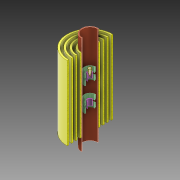
# Autodesk Inventor part: DemoCrossSect
Saved by Autodesk Inventor 2021 (Build 250183000, 183)
## iProperties
Created: 2023-01-16
Part Number: DemoCrossSect
Material: Copper
Document SubType Name: Modeling
Designer: Eli
Density: 8.94 g/cm^3
Appearance: Copper - Satin
Author: Eli
Autodesk Inventor part; units mm, degrees
ref_plane "YZ Plane" through (0, 0, 0) normal (1, 0, 0) x (0, 1, 0)
ref_plane "XZ Plane" through (0, 0, 0) normal (0, 1, 0) x (-1, 0, 0)
ref_plane "XY Plane" through (0, 0, 0) normal (0, 0, 1) x (1, 0, 0)
sketch "Sketch1" plane through (0, 0, 0) normal (0, 0, 1) x (1, 0, 0)
  line L0 (18.1725, 115.942) -> (19.9396, 115.942)
  line L1 (19.9396, 115.942) -> (19.9396, 77.2947)
  line L2 (19.9396, -115.942) -> (18.1725, -115.942)
  line L3 (18.1725, -115.942) -> (18.1725, 115.942)
  line L4 (19.9396, 77.2947) -> (19.9396, -77.2947)
  line L5 (19.9396, -77.2947) -> (19.9396, -115.942)
  line L6 (27.9401, -86.9565) -> (30.8386, -86.9565)
  line L7 (0, 289.8551) -> (0, -289.8551)
  line L8 (0, 57.971) -> (0, -57.971)
  line L9 (5.314, 35.2657) -> (6.2802, 35.2657)
  line L10 (5.314, 20.7729) -> (6.2802, 20.7729)
  line L11 (5.314, 35.2657) -> (5.314, 20.7729)
  line L12 (6.2802, 20.7729) -> (6.2802, 35.2657)
  arc A0 (0, -289.8551) -> (0, 289.8551) centre (0, 0) ccw
  arc A1 (9.6618, 30.9179) -> (11.6908, 30.9179) centre (10.6763, 30.9179) ccw
  arc A2 (11.6908, 30.9179) -> (9.6618, 30.9179) centre (10.6763, 30.9179) ccw
  arc A3 (9.6618, 32.9952) -> (11.6908, 32.9952) centre (10.6763, 32.9952) ccw
  arc A4 (11.6908, 32.9952) -> (9.6618, 32.9952) centre (10.6763, 32.9952) ccw
  arc A5 (9.6618, 35.0725) -> (11.6908, 35.0725) centre (10.6763, 35.0725) ccw
  arc A6 (11.6908, 35.0725) -> (9.6618, 35.0725) centre (10.6763, 35.0725) ccw
  arc A7 (9.6618, 37.1498) -> (11.6908, 37.1498) centre (10.6763, 37.1498) ccw
  arc A8 (11.6908, 37.1498) -> (9.6618, 37.1498) centre (10.6763, 37.1498) ccw
  arc A9 (9.6618, 39.2271) -> (11.6908, 39.2271) centre (10.6763, 39.2271) ccw
  arc A10 (11.6908, 39.2271) -> (9.6618, 39.2271) centre (10.6763, 39.2271) ccw
  arc A11 (9.6618, 41.3043) -> (11.6908, 41.3043) centre (10.6763, 41.3043) ccw
  arc A12 (11.6908, 41.3043) -> (9.6618, 41.3043) centre (10.6763, 41.3043) ccw
  arc A13 (11.4976, 31.9614) -> (13.5266, 31.9614) centre (12.5121, 31.9614) ccw
  arc A14 (13.5266, 31.9614) -> (11.4976, 31.9614) centre (12.5121, 31.9614) ccw
  arc A15 (11.4976, 34.0386) -> (13.5266, 34.0386) centre (12.5121, 34.0386) ccw
  arc A16 (13.5266, 34.0386) -> (11.4976, 34.0386) centre (12.5121, 34.0386) ccw
  arc A17 (11.4976, 36.1159) -> (13.5266, 36.1159) centre (12.5121, 36.1159) ccw
  arc A18 (13.5266, 36.1159) -> (11.4976, 36.1159) centre (12.5121, 36.1159) ccw
  arc A19 (11.4976, 38.1932) -> (13.5266, 38.1932) centre (12.5121, 38.1932) ccw
  arc A20 (13.5266, 38.1932) -> (11.4976, 38.1932) centre (12.5121, 38.1932) ccw
  arc A21 (11.4976, 40.2705) -> (13.5266, 40.2705) centre (12.5121, 40.2705) ccw
  arc A22 (13.5266, 40.2705) -> (11.4976, 40.2705) centre (12.5121, 40.2705) ccw
  arc A23 (11.6908, 25.1208) -> (9.6618, 25.1208) centre (10.6763, 25.1208) ccw
  arc A24 (9.6618, 25.1208) -> (11.6908, 25.1208) centre (10.6763, 25.1208) ccw
  arc A25 (11.6908, 23.0435) -> (9.6618, 23.0435) centre (10.6763, 23.0435) ccw
  arc A26 (9.6618, 23.0435) -> (11.6908, 23.0435) centre (10.6763, 23.0435) ccw
  arc A27 (11.6908, 20.9662) -> (9.6618, 20.9662) centre (10.6763, 20.9662) ccw
  arc A28 (9.6618, 20.9662) -> (11.6908, 20.9662) centre (10.6763, 20.9662) ccw
  arc A29 (11.6908, 18.8889) -> (9.6618, 18.8889) centre (10.6763, 18.8889) ccw
  arc A30 (9.6618, 18.8889) -> (11.6908, 18.8889) centre (10.6763, 18.8889) ccw
  arc A31 (11.6908, 16.8116) -> (9.6618, 16.8116) centre (10.6763, 16.8116) ccw
  arc A32 (9.6618, 16.8116) -> (11.6908, 16.8116) centre (10.6763, 16.8116) ccw
  arc A33 (11.6908, 14.7343) -> (9.6618, 14.7343) centre (10.6763, 14.7343) ccw
  arc A34 (9.6618, 14.7343) -> (11.6908, 14.7343) centre (10.6763, 14.7343) ccw
  arc A35 (13.5266, 24.0773) -> (11.4976, 24.0773) centre (12.5121, 24.0773) ccw
  arc A36 (11.4976, 24.0773) -> (13.5266, 24.0773) centre (12.5121, 24.0773) ccw
  arc A37 (13.5266, 22) -> (11.4976, 22) centre (12.5121, 22) ccw
  arc A38 (11.4976, 22) -> (13.5266, 22) centre (12.5121, 22) ccw
  arc A39 (13.5266, 19.9227) -> (11.4976, 19.9227) centre (12.5121, 19.9227) ccw
  arc A40 (11.4976, 19.9227) -> (13.5266, 19.9227) centre (12.5121, 19.9227) ccw
  arc A41 (13.5266, 17.8454) -> (11.4976, 17.8454) centre (12.5121, 17.8454) ccw
  arc A42 (11.4976, 17.8454) -> (13.5266, 17.8454) centre (12.5121, 17.8454) ccw
  arc A43 (13.5266, 15.7681) -> (11.4976, 15.7681) centre (12.5121, 15.7681) ccw
  arc A44 (11.4976, 15.7681) -> (13.5266, 15.7681) centre (12.5121, 15.7681) ccw
  arc A45 (11.6908, -30.9179) -> (9.6618, -30.9179) centre (10.6763, -30.9179) ccw
  arc A46 (9.6618, -30.9179) -> (11.6908, -30.9179) centre (10.6763, -30.9179) ccw
  arc A47 (11.6908, -32.9952) -> (9.6618, -32.9952) centre (10.6763, -32.9952) ccw
  arc A48 (9.6618, -32.9952) -> (11.6908, -32.9952) centre (10.6763, -32.9952) ccw
  arc A49 (11.6908, -35.0725) -> (9.6618, -35.0725) centre (10.6763, -35.0725) ccw
  arc A50 (9.6618, -35.0725) -> (11.6908, -35.0725) centre (10.6763, -35.0725) ccw
  arc A51 (11.6908, -37.1498) -> (9.6618, -37.1498) centre (10.6763, -37.1498) ccw
  arc A52 (9.6618, -37.1498) -> (11.6908, -37.1498) centre (10.6763, -37.1498) ccw
  arc A53 (11.6908, -39.2271) -> (9.6618, -39.2271) centre (10.6763, -39.2271) ccw
  arc A54 (9.6618, -39.2271) -> (11.6908, -39.2271) centre (10.6763, -39.2271) ccw
  arc A55 (11.6908, -41.3043) -> (9.6618, -41.3043) centre (10.6763, -41.3043) ccw
  arc A56 (9.6618, -41.3043) -> (11.6908, -41.3043) centre (10.6763, -41.3043) ccw
  arc A57 (13.5266, -31.9614) -> (11.4976, -31.9614) centre (12.5121, -31.9614) ccw
  arc A58 (11.4976, -31.9614) -> (13.5266, -31.9614) centre (12.5121, -31.9614) ccw
  arc A59 (13.5266, -34.0386) -> (11.4976, -34.0386) centre (12.5121, -34.0386) ccw
  arc A60 (11.4976, -34.0386) -> (13.5266, -34.0386) centre (12.5121, -34.0386) ccw
  arc A61 (13.5266, -36.1159) -> (11.4976, -36.1159) centre (12.5121, -36.1159) ccw
  arc A62 (11.4976, -36.1159) -> (13.5266, -36.1159) centre (12.5121, -36.1159) ccw
  arc A63 (13.5266, -38.1932) -> (11.4976, -38.1932) centre (12.5121, -38.1932) ccw
  arc A64 (11.4976, -38.1932) -> (13.5266, -38.1932) centre (12.5121, -38.1932) ccw
  arc A65 (13.5266, -40.2705) -> (11.4976, -40.2705) centre (12.5121, -40.2705) ccw
  arc A66 (11.4976, -40.2705) -> (13.5266, -40.2705) centre (12.5121, -40.2705) ccw
  arc A67 (9.6618, -25.1208) -> (11.6908, -25.1208) centre (10.6763, -25.1208) ccw
  arc A68 (11.6908, -25.1208) -> (9.6618, -25.1208) centre (10.6763, -25.1208) ccw
  arc A69 (9.6618, -23.0435) -> (11.6908, -23.0435) centre (10.6763, -23.0435) ccw
  arc A70 (11.6908, -23.0435) -> (9.6618, -23.0435) centre (10.6763, -23.0435) ccw
  arc A71 (9.6618, -20.9662) -> (11.6908, -20.9662) centre (10.6763, -20.9662) ccw
  arc A72 (11.6908, -20.9662) -> (9.6618, -20.9662) centre (10.6763, -20.9662) ccw
  arc A73 (9.6618, -18.8889) -> (11.6908, -18.8889) centre (10.6763, -18.8889) ccw
  arc A74 (11.6908, -18.8889) -> (9.6618, -18.8889) centre (10.6763, -18.8889) ccw
  arc A75 (9.6618, -16.8116) -> (11.6908, -16.8116) centre (10.6763, -16.8116) ccw
  arc A76 (11.6908, -16.8116) -> (9.6618, -16.8116) centre (10.6763, -16.8116) ccw
  arc A77 (9.6618, -14.7343) -> (11.6908, -14.7343) centre (10.6763, -14.7343) ccw
  arc A78 (11.6908, -14.7343) -> (9.6618, -14.7343) centre (10.6763, -14.7343) ccw
  arc A79 (11.4976, -24.0773) -> (13.5266, -24.0773) centre (12.5121, -24.0773) ccw
  arc A80 (13.5266, -24.0773) -> (11.4976, -24.0773) centre (12.5121, -24.0773) ccw
  arc A81 (11.4976, -22) -> (13.5266, -22) centre (12.5121, -22) ccw
  arc A82 (13.5266, -22) -> (11.4976, -22) centre (12.5121, -22) ccw
  arc A83 (11.4976, -19.9227) -> (13.5266, -19.9227) centre (12.5121, -19.9227) ccw
  arc A84 (13.5266, -19.9227) -> (11.4976, -19.9227) centre (12.5121, -19.9227) ccw
  arc A85 (11.4976, -17.8454) -> (13.5266, -17.8454) centre (12.5121, -17.8454) ccw
  arc A86 (13.5266, -17.8454) -> (11.4976, -17.8454) centre (12.5121, -17.8454) ccw
  arc A87 (11.4976, -15.7681) -> (13.5266, -15.7681) centre (12.5121, -15.7681) ccw
  arc A88 (13.5266, -15.7681) -> (11.4976, -15.7681) centre (12.5121, -15.7681) ccw
  line L13 (19.9396, 86.9565) -> (23.9396, 86.9565)
  line L14 (23.9396, 86.9565) -> (23.9396, -86.9565)
  line L15 (23.9396, -86.9565) -> (19.9396, -86.9565)
  line L16 (19.9396, -86.9565) -> (19.9396, 86.9565)
  line L17 (29.9396, 86.9565) -> (33.9396, 86.9565)
  line L18 (29.9396, -86.9565) -> (29.9396, 86.9565)
  line L19 (33.9396, 86.9565) -> (33.9396, -86.9565)
  line L20 (33.9396, -86.9565) -> (29.9396, -86.9565)
  line L21 (39.9396, 86.9565) -> (43.9396, 86.9565)
  line L22 (39.9396, -86.9565) -> (39.9396, 86.9565)
  line L23 (43.9396, 86.9565) -> (43.9396, -86.9565)
  line L24 (43.9396, -86.9565) -> (39.9396, -86.9565)
  line L25 (49.9396, 86.9565) -> (53.9396, 86.9565)
  line L26 (49.9396, -86.9565) -> (49.9396, 86.9565)
  line L27 (53.9396, 86.9565) -> (53.9396, -86.9565)
  line L28 (53.9396, -86.9565) -> (49.9396, -86.9565)
  line L29 (0, 23.6243) -> (4, 38.6243)
  line L30 (4, 38.6243) -> (4, 44.6243)
  line L31 (4, 44.6243) -> (0, 44.6243)
  line L32 (0, 23.6243) -> (0, 44.6243)
  line L33 (0, -405.7971) -> (0, 405.7971) projected
  line L34 (1.1854, 28.0696) -> (0, 28.0696) construction
  arc A89 (0, 28.0696) -> (1.4909, 29.215) centre (0, 29.6126) ccw
  point P0 (9.6618, 41.3043)
  point P1 (11.6908, 41.3043)
  point P2 (11.4976, 40.2705)
  point P3 (13.5266, 40.2705)
  point P4 (9.6618, 39.2271)
  point P5 (11.6908, 39.2271)
  point P6 (11.4976, 38.1932)
  point P7 (13.5266, 38.1932)
  point P8 (9.6618, 37.1498)
  point P9 (11.6908, 37.1498)
  point P10 (9.6618, 35.0725)
  point P11 (11.6908, 35.0725)
  point P12 (11.4976, 36.1159)
  point P13 (13.5266, 36.1159)
  point P14 (11.4976, 34.0386)
  point P15 (13.5266, 34.0386)
  point P16 (9.6618, 32.9952)
  point P17 (11.6908, 32.9952)
  point P18 (11.4976, 31.9614)
  point P19 (13.5266, 31.9614)
  point P20 (9.6618, 30.9179)
  point P21 (11.6908, 30.9179)
  point P22 (11.6908, 25.1208)
  point P23 (9.6618, 25.1208)
  point P24 (13.5266, 24.0773)
  point P25 (11.4976, 24.0773)
  point P26 (11.6908, 23.0435)
  point P27 (9.6618, 23.0435)
  point P28 (13.5266, 22)
  point P29 (11.4976, 22)
  point P30 (11.6908, 20.9662)
  point P31 (9.6618, 20.9662)
  point P32 (13.5266, 19.9227)
  point P33 (11.4976, 19.9227)
  point P34 (11.6908, 18.8889)
  point P35 (9.6618, 18.8889)
  point P36 (13.5266, 17.8454)
  point P37 (11.4976, 17.8454)
  point P38 (11.6908, 16.8116)
  point P39 (9.6618, 16.8116)
  point P40 (13.5266, 15.7681)
  point P41 (11.4976, 15.7681)
  point P42 (11.6908, 14.7343)
  point P43 (9.6618, 14.7343)
  point P44 (0, 44.6243)
  point P45 (0, 23.6243)
  point P46 (0, 28.0696)
  dimension "d3" = 4
  dimension "d6" = 10
  dimension "d12" = 4
  dimension "d13" = 15
  dimension "d14" = 6
  constraints: 180 point on circle, 90 centre point, 68 end point, 6 point on line, 3 collinear, 3 perpendicular, 2 horizontal, 2 parallel, 2 tangent, 1 vertical, 23 other
  measures "d3" distance of L14.end L15.end
  measures "d6" distance of L13.start L17.start
  measures "d12" distance between parallel lines of L8 L30
  measures "d13" vertical distance of L29.start L29.end
  measures "d14" distance of L29.end L30.end
revolve "Revolution1" add sketch "Sketch1" angle 360 about axis through (0, 289.8551, 0) along (0, -1, 0) contours A2 A1 | A4 A3 | A6 A5 | A8 A7 | A10 A9 | A12 A11 | A14 A13 | A16 A15 | A18 A17 | A20 A19 | A22 A21 | A24 A23 | A26 A25 | A28 A27 | A30 A29 | A32 A31 | A34 A33 | A36 A35 | A38 A37 | A40 A39 | A42 A41 | A44 A43
revolve "Revolution2" add sketch "Sketch1" angle 360 about axis through (0, 57.971, 0) along (0, -1, 0) separate body contours L9 L12 L10 L11
revolve "Revolution3" add sketch "Sketch1" angle 360 about axis through (0, 57.971, 0) along (0, -1, 0) separate body contours L0 L1 L4 L5 L2 L3
revolve "Revolution4" add sketch "Sketch1" angle 360 about axis through (0, 289.8551, 0) along (0, -1, 0) separate body contours L13 L14 L15 L5 L4 L1 | L18 L17 L19 L20 L6 | L21 L23 L24 L22 | L25 L27 L28 L26
mirror "Mirror1" about plane through (0, 0, 0) normal (0, 1, 0) bodies 2 1
revolve "Revolution5" add sketch "Sketch1" angle 360 about axis through (0, -10, 0) along (0, 1, 0) separate body contours L31 L30 L29 A89 L7
shell "Shell1" thickness 0.25 removed faces 1 at (0.998, 44.6243, -0.8842) bodies 5
sketch "Sketch2" plane through (0, 0, 0) normal (0, 0, 1) x (1, 0, 0)
  line L0 (-4, 44.6243) -> (-4, 38.6243) projected
  line L1 (-4, 38.6243) -> (-1.4909, 29.215) projected
  arc A0 (-1.2493, 29.2794) -> (1.2493, 29.2794) centre (0, 29.6126) ccw projected
  line L2 (-3.75, 38.657) -> (-1.2493, 29.2794) projected
  line L3 (3.75, 38.657) -> (1.2493, 29.2794) projected
  line L4 (0, 28.3196) -> (0, 30.173)
  line L5 (0, 30.173) -> (1.4876, 30.173)
  point P0 (0, 0)
  constraints: 4 end point, 1 perpendicular, 1 point on circle, 1 point on line, 1 vertical
revolve "Revolution6" add sketch "Sketch2" angle 360 about axis through (0, 28.3196, 0) along (0, 1, 0) separate body
body "Solid1"
body "Solid2"
body "Solid3"
body "Solid4"
body "Solid5"
body "Solid6"
